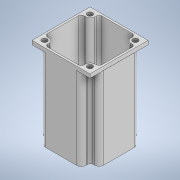
# Autodesk Inventor part: NEMA23_Shroud
Saved by Autodesk Inventor 2021 (Build 250183000, 183)
## iProperties
Created: 2021-03-31
Part Number: NEMA23_Shroud
Material: Generic
Document SubType Name: Modeling
Designer: Jorian Brusind
Density: 1 g/cm^3
Appearance: Default
Author: Jorian Brusind
Autodesk Inventor part; units mm, degrees
ref_plane "YZ Plane" through (0, 0, 0) normal (1, 0, 0) x (0, 1, 0)
ref_plane "XZ Plane" through (0, 0, 0) normal (0, 1, 0) x (-1, 0, 0)
ref_plane "XY Plane" through (0, 0, 0) normal (0, 0, 1) x (1, 0, 0)
ref_plane "Work Plane1" through (0, 3, 0) normal (0, 1, 0) x (1, 0, 0)
sketch "Sketch2" plane through (0, 3, 0) normal (0, 1, 0) x (1, 0, 0)
  line L0 (0, 12.2943) -> (0, 43.7057)
  arc A0 (-3.0277, 9.4339) -> (0, 12.2943) centre (-2.9968, 12.4338) ccw
  line L1 (-4.5807, 9.4339) -> (-3.0277, 9.4339)
  arc A1 (-4.5807, 9.4339) -> (-9.0279, 4.4646) centre (-4.0279, 4.4646) ccw
  line L2 (-9.0279, 2.9638) -> (-9.0279, 4.4646)
  arc A2 (-12.0277, 0) -> (-9.0279, 2.9638) centre (-12.0277, 3) ccw
  line L3 (-44.022, 0) -> (-12.0277, 0)
  arc A3 (-46.5576, 2.9638) -> (-44.022, 0) centre (-43.5576, 2.9638) ccw
  line L4 (-46.5576, 4.5169) -> (-46.5576, 2.9638)
  arc A4 (-46.5576, 4.5169) -> (-51.5269, 8.9638) centre (-51.5269, 3.9638) ccw
  line L5 (-53.0277, 8.9638) -> (-51.5269, 8.9638)
  arc A5 (-56, 11.5573) -> (-53.0277, 8.9638) centre (-53.0277, 11.9638) ccw
  line L6 (-56, 44.3704) -> (-56, 11.5573)
  arc A6 (-53.0277, 46.9638) -> (-56, 44.3704) centre (-53.0277, 43.9638) ccw
  arc A7 (-51.5269, 46.9638) -> (-46.5576, 51.4108) centre (-51.5269, 51.9638) ccw
  line L7 (-51.5269, 46.9638) -> (-53.0277, 46.9638)
  arc A8 (-43.5578, 56) -> (-46.5576, 52.9638) centre (-43.5578, 53) ccw
  line L8 (-46.5576, 52.9638) -> (-46.5576, 51.4108)
  line L9 (-12.0277, 56) -> (-43.5578, 56)
  arc A9 (-9.0277, 53) -> (-12.0277, 56) centre (-12.0277, 53) ccw
  line L10 (-9.0277, 51.4993) -> (-9.0277, 53)
  arc A10 (-9.0277, 51.4993) -> (-4.5807, 46.5299) centre (-4.0277, 51.4993) ccw
  line L11 (-3.0277, 46.5299) -> (-4.5807, 46.5299)
  arc A11 (0, 43.7057) -> (-3.0277, 46.5299) centre (-2.9949, 43.5301) ccw
  arc A12 (-43.5578, 58) -> (-48.5576, 52.9533) centre (-43.5578, 53) ccw
  line L12 (-48.5576, 52.9533) -> (-48.5576, 51.5359)
  arc A13 (-51.5269, 48.9638) -> (-48.5576, 51.5359) centre (-51.5269, 51.9638) ccw
  line L13 (-51.5269, 48.9638) -> (-53.0277, 48.9638)
  arc A14 (-53.0277, 48.9638) -> (-58, 44.4892) centre (-53.0277, 43.9638) ccw
  line L14 (-58, 44.4892) -> (-58, 11.4385)
  arc A15 (-58, 11.4385) -> (-53.0277, 6.9638) centre (-53.0277, 11.9638) ccw
  line L15 (-53.0277, 6.9638) -> (-51.5269, 6.9638)
  arc A16 (-48.5576, 4.3918) -> (-51.5269, 6.9638) centre (-51.5269, 3.9638) ccw
  line L16 (-48.5576, 4.3918) -> (-48.5576, 2.9638)
  arc A17 (-48.5576, 2.9638) -> (-44.1579, -2) centre (-43.5576, 2.9638) ccw
  line L17 (-44.1579, -2) -> (-12.0277, -2)
  arc A18 (-12.0277, -2) -> (-7.0279, 2.9533) centre (-12.0277, 3) ccw
  line L18 (-7.0279, 2.9533) -> (-7.0279, 4.4646)
  arc A19 (-4.4557, 7.4339) -> (-7.0279, 4.4646) centre (-4.0279, 4.4646) ccw
  line L19 (-4.4557, 7.4339) -> (-3.0367, 7.4339)
  arc A20 (-3.0367, 7.4339) -> (2, 12.2537) centre (-2.9968, 12.4338) ccw
  line L20 (2, 12.2537) -> (2, 43.7568)
  arc A21 (2, 43.7568) -> (-3.0372, 48.5299) centre (-2.9949, 43.5301) ccw
  line L21 (-3.0372, 48.5299) -> (-4.4556, 48.5299)
  arc A22 (-7.0277, 51.4993) -> (-4.4556, 48.5299) centre (-4.0277, 51.4993) ccw
  line L22 (-7.0277, 51.4993) -> (-7.0277, 53)
  arc A23 (-7.0277, 53) -> (-12.0277, 58) centre (-12.0277, 53) ccw
  line L23 (-12.0277, 58) -> (-43.5578, 58)
  line L24 (0, 0) -> (-56, 0)
  line L25 (0, 0) -> (0, 56)
  dimension "d17" = 5
  dimension "d18" = 5
  dimension "d19" = 5
  dimension "d20" = 5
  dimension "d24" = 2
  dimension "d28" = 56
  dimension "d29" = 56
  constraints: 52 end point, 48 point on circle, 24 centre point, 2 point on line, 23 other
  measures "d17" radius of A7
  measures "d18" radius of A4
  measures "d19" radius of A1
  measures "d20" radius of A10
  measures "d24" distance between parallel lines of L9 L23
  measures "d28" distance of L24.start L24.end
  measures "d29" distance of L24.start L25.end
extrude "Extrusion2" add sketch "Sketch2" along normal blind 89 contours L25 A20 L19 A19 L18 A18 L24 A2 L2 A1 L1 A0 | L0 L25 A21 L20 A20 | A11 L11 A10 L10 A9 L9 A8 L8 A7 L7 A6 L6 A5 L5 A4 L4 A3 L24 A17 L16 A16 L15 A15 L14 A14 L13 A13 L12 A12 L23 A23 L22 A22 L21 A21 L25 | A18 L17 A17 L24 L3
sketch "Sketch3" plane through (0, 3, 0) normal (0, -1, 0) x (1, 0, 0)
  line L0 (0, -43.7057) -> (0, -12.2943) projected
  line L1 (0, -12.2943) -> (0, -43.7057)
  line L2 (-43.5578, -56) -> (-12.0277, -56) projected
  arc A0 (-12.0277, -56) -> (-9.0277, -53) centre (-12.0277, -53) ccw projected
  arc A1 (-4.5807, -46.5299) -> (-9.0277, -51.4993) centre (-4.0277, -51.4993) ccw projected
  line L3 (-9.0277, -53) -> (-9.0277, -51.4993) projected
  arc A2 (-3.0277, -46.5299) -> (0, -43.7057) centre (-2.9949, -43.5301) ccw projected
  line L4 (-4.5807, -46.5299) -> (-3.0277, -46.5299) projected
  arc A3 (-46.5576, -52.9638) -> (-43.5578, -56) centre (-43.5578, -53) ccw projected
  arc A4 (-46.5576, -51.4108) -> (-51.5269, -46.9638) centre (-51.5269, -51.9638) ccw projected
  line L5 (-46.5576, -51.4108) -> (-46.5576, -52.9638) projected
  arc A5 (-56, -44.3704) -> (-53.0277, -46.9638) centre (-53.0277, -43.9638) ccw projected
  line L6 (-53.0277, -46.9638) -> (-51.5269, -46.9638) projected
  line L7 (-56, -11.5573) -> (-56, -44.3704) projected
  arc A6 (-53.0277, -8.9638) -> (-56, -11.5573) centre (-53.0277, -11.9638) ccw projected
  line L8 (-51.5269, -8.9638) -> (-53.0277, -8.9638) projected
  arc A7 (-51.5269, -8.9638) -> (-46.5576, -4.5169) centre (-51.5269, -3.9638) ccw projected
  arc A8 (-44.022, 0) -> (-46.5576, -2.9638) centre (-43.5576, -2.9638) ccw projected
  line L9 (-12.0277, 0) -> (-44.022, 0) projected
  line L10 (-46.5576, -2.9638) -> (-46.5576, -4.5169) projected
  arc A9 (-9.0279, -2.9638) -> (-12.0277, 0) centre (-12.0277, -3) ccw projected
  line L11 (-9.0279, -4.4646) -> (-9.0279, -2.9638) projected
  arc A10 (-9.0279, -4.4646) -> (-4.5807, -9.4339) centre (-4.0279, -4.4646) ccw projected
  line L12 (-3.0277, -9.4339) -> (-4.5807, -9.4339) projected
  arc A11 (0, -12.2943) -> (-3.0277, -9.4339) centre (-2.9968, -12.4338) ccw projected
  point P0 (0, 0)
  constraints: 2 end point, 1 collinear
extrude "Extrusion3" add sketch "Sketch3" against normal blind 3
sketch "Sketch4" plane through (0, 92, 0) normal (0, 1, 0) x (1, 0, 0)
  line L0 (2, 12.2537) -> (2, 43.7568) projected
  line L1 (2, 28.0053) -> (-58, 27.9638)
  line L2 (-58, 44.4892) -> (-58, 11.4385) projected
  line L3 (-12.0277, 58) -> (-43.5578, 58) projected
  line L4 (-27.7928, 58) -> (-28.0928, -2)
  line L5 (-44.1579, -2) -> (-12.0277, -2) projected
  line L6 (2.0572, 58) -> (-57.9428, 58)
  line L7 (-57.9428, 58) -> (-57.9428, -2)
  line L8 (-57.9428, -2) -> (2.0572, -2)
  line L9 (2.0572, -2) -> (2.0572, 58)
  line L10 (2.0572, 58) -> (-57.9428, -2) construction
  line L11 (-57.9428, 58) -> (2.0572, -2) construction
  arc A0 (-4.4557, 7.4339) -> (-7.0279, 4.4646) centre (-4.0279, 4.4646) ccw projected
  line L12 (-7.0279, 2.9533) -> (-7.0279, 4.4646) projected
  arc A1 (-12.0277, -2) -> (-7.0279, 2.9533) centre (-12.0277, 3) ccw projected
  arc A2 (-3.0367, 7.4339) -> (2, 12.2537) centre (-2.9968, 12.4338) ccw projected
  line L13 (-4.4557, 7.4339) -> (-3.0367, 7.4339) projected
  arc A3 (2, 43.7568) -> (-3.0372, 48.5299) centre (-2.9949, 43.5301) ccw projected
  line L14 (-3.0372, 48.5299) -> (-4.4556, 48.5299) projected
  arc A4 (-7.0277, 51.4993) -> (-4.4556, 48.5299) centre (-4.0277, 51.4993) ccw projected
  line L15 (-7.0277, 51.4993) -> (-7.0277, 53) projected
  arc A5 (-7.0277, 53) -> (-12.0277, 58) centre (-12.0277, 53) ccw projected
  arc A6 (-43.5578, 58) -> (-48.5576, 52.9533) centre (-43.5578, 53) ccw projected
  line L16 (-48.5576, 52.9533) -> (-48.5576, 51.5359) projected
  arc A7 (-51.5269, 48.9638) -> (-48.5576, 51.5359) centre (-51.5269, 51.9638) ccw projected
  line L17 (-51.5269, 48.9638) -> (-53.0277, 48.9638) projected
  arc A8 (-53.0277, 48.9638) -> (-58, 44.4892) centre (-53.0277, 43.9638) ccw projected
  arc A9 (-58, 11.4385) -> (-53.0277, 6.9638) centre (-53.0277, 11.9638) ccw projected
  line L18 (-53.0277, 6.9638) -> (-51.5269, 6.9638) projected
  arc A10 (-48.5576, 4.3918) -> (-51.5269, 6.9638) centre (-51.5269, 3.9638) ccw projected
  line L19 (-48.5576, 4.3918) -> (-48.5576, 2.9638) projected
  arc A11 (-48.5576, 2.9638) -> (-44.1579, -2) centre (-43.5576, 2.9638) ccw projected
  point P0 (0, 0)
  point P1 (-27.9428, 28)
  point P2 (-57.9428, 44.8814)
  point P3 (-57.9428, 11.0463)
  point P4 (-44.1579, -2)
  dimension "d64" = 60
  dimension "d65" = 60
  constraints: 16 end point, 7 midpoint, 2 parallel, 1 horizontal, 1 perpendicular
  measures "d64" distance of L8.end L7.end
  measures "d65" distance of L7.end L6.end
extrude "Extrusion7" add sketch "Sketch4" against normal blind 4 contours L0 A3 L14 A4 L15 A5 L6 L9 L8 A1 L12 A0 L13 A2 | L7 L6 A6 L16 A7 L17 A8 | A9 L18 A10 L19 A11 L8 L7
sketch "Sketch7" plane through (0, 88, 0) normal (0, -1, 0) x (1, 0, 0)
  circle A0 centre (-4.5, -4.5) radius 2.75
  line L0 (-12.0277, 0) -> (-44.022, 0) projected
  line L1 (0, -43.7057) -> (0, -12.2943) projected
  line L2 (-44.022, 0) -> (-12.0277, 0)
  line L3 (-56, -11.5573) -> (-56, -44.3704) projected
  line L4 (-56, -11.5573) -> (-56, -44.3704)
  circle A1 centre (-51.5, -4.5) radius 2.75
  circle A2 centre (-4.5, -51.5) radius 2.75
  circle A3 centre (-51.5, -51.5) radius 2.75
  point P0 (0, 0)
  dimension "d68" = 5.5
  dimension "d69" = 4.5
  dimension "d70" = 4.5
  dimension "d73" = 47
  dimension "d76" = 47
  constraints: 4 centre point, 4 end point, 2 vertical, 1 collinear, 1 horizontal, 6 other
  measures "d68" diameter of A0
  measures "d69" distance from line of L0 A0.centre
  measures "d70" distance from line of L1 A0.centre
  measures "d73" distance of A0.centre A1.centre
  measures "d76" distance of A0.centre A2.centre
extrude "Extrusion8" cut sketch "Sketch7" against normal blind 4
body "Solid1"
